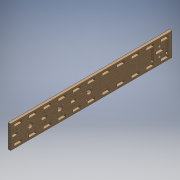
# Autodesk Inventor part: BearingMotorColumn
Saved by Autodesk Inventor 2016 (Build 200138000, 138)
## iProperties
Created: 2015-11-25
Part Number: BearingMotorColumn
Material: MDF Medium Density Fiberboard
Document SubType Name: Modeling
Designer: momem
Density: 0.8 g/cm^3
Appearance: Cardboard - Corrugated
MotorWidth: 37.000 mm
SupportClearance: 5.000 mm
MotorShaftWidth: 12.000 mm
CouplingWidth: 0.375 in
CouplingDiameter: 0.870 in
DiskGap: 75.835 mm
d28: 360.00 deg
ColumnWidth: 59.780 mm
WoodThickness: 6.390 mm
ColumnHeight: 417.094 mm
BearingDiameter: 24.000 mm
BearingWidth: 7.000 mm
BearingShaftDiameter: 8.000 mm
ZipTieWidth: 2.500 mm
ZipTieThickness: 1.100 mm
ZipTieClearance: 1.000 mm
ZipTieDistance: 10.000 mm
BearingHolderHeight: 13.100 mm
ZipTieHorDistance: 21.100 mm
ZipTieVerDistance: 9.500 mm
d97: 63.266 mm
d98: 227.506 mm
MotorWheel: 45.445 mm
BearingShaftOffset: 1.574 mm
BearingHolderHeight_1: 23.674 mm
LatchHeight: 13.147 mm
d176: 34.539 mm
Author: momem
Autodesk Inventor part; units mm, degrees
ref_plane "YZ Plane" through (0, 0, 0) normal (1, 0, 0) x (0, 1, 0)
ref_plane "XZ Plane" through (0, 0, 0) normal (0, 1, 0) x (-1, 0, 0)
ref_plane "XY Plane" through (0, 0, 0) normal (0, 0, 1) x (1, 0, 0)
sketch "Sketch1" plane through (0, 0, 0) normal (1, 0, 0) x (0, 1, 0)
  line L0 (37.9177, 29.89) -> (-37.9177, 29.89)
  line L1 (-37.9177, 29.89) -> (-37.9177, -29.89)
  line L2 (-37.9177, -29.89) -> (37.9177, -29.89)
  line L3 (37.9177, -29.89) -> (37.9177, 29.89) construction
  circle A0 centre (13.7687, 0) radius 6
  line L4 (-20.7703, 3.163) -> (-33.9177, 3.163)
  line L5 (-33.9177, 3.163) -> (-33.9177, -3.163)
  line L6 (-33.9177, -3.163) -> (-20.7703, -3.163)
  line L7 (-20.7703, -3.163) -> (-20.7703, 3.163)
  circle A1 centre (13.7687, 0) radius 11.049 construction
  circle A2 centre (6.7687, 0) radius 18.5 construction
  line L8 (28.4382, 24.8261) -> (9.4794, 24.8261)
  line L9 (9.4794, 24.8261) -> (9.4794, 18.5)
  line L10 (9.4794, 18.5) -> (28.4382, 18.5)
  line L11 (28.4382, 18.5) -> (28.4382, 24.8261)
  line L12 (-9.4794, 18.5) -> (-9.4794, 24.8261)
  line L13 (-9.4794, 24.8261) -> (-28.4382, 24.8261)
  line L14 (-28.4382, 18.5) -> (-9.4794, 18.5)
  line L15 (-28.4382, 24.8261) -> (-28.4382, 18.5)
  line L16 (28.4382, -24.89) -> (28.4382, -18.5639)
  line L17 (28.4382, -18.5639) -> (9.4794, -18.5639)
  line L18 (9.4794, -24.89) -> (28.4382, -24.89)
  line L19 (9.4794, -18.5639) -> (9.4794, -24.89)
  line L20 (-9.4794, -24.89) -> (-9.4794, -18.5639)
  line L21 (-9.4794, -18.5639) -> (-28.4382, -18.5639)
  line L22 (-28.4382, -24.89) -> (-9.4794, -24.89)
  line L23 (-28.4382, -18.5639) -> (-28.4382, -24.89)
  circle A3 centre (6.7687, -15.5) radius 1.5
  circle A4 centre (20.1921, -7.75) radius 1.5
  circle A5 centre (20.1921, 7.75) radius 1.5
  circle A6 centre (6.7687, 15.5) radius 1.5
  circle A7 centre (-6.6547, 7.75) radius 1.5
  circle A8 centre (-6.6547, -7.75) radius 1.5
  line L24 (-22.7703, 11.1) -> (-25.2703, 11.1)
  line L25 (-25.2703, 11.1) -> (-25.2703, 10)
  line L26 (-25.2703, 10) -> (-22.7703, 10)
  line L27 (-22.7703, 10) -> (-22.7703, 11.1)
  line L28 (-27.344, 3.1631) -> (-27.344, -3.1631) construction
  line L29 (-20.7703, 0) -> (-33.9177, 0) construction
  line L30 (-31.9177, 11.1) -> (-29.4177, 11.1)
  line L31 (-29.4177, 11.1) -> (-29.4177, 10)
  line L32 (-29.4177, 10) -> (-31.9177, 10)
  line L33 (-31.9177, 10) -> (-31.9177, 11.1)
  line L34 (-22.7703, -11.1) -> (-25.2703, -11.1)
  line L35 (-25.2703, -11.1) -> (-25.2703, -10)
  line L36 (-25.2703, -10) -> (-22.7703, -10)
  line L37 (-22.7703, -10) -> (-22.7703, -11.1)
  line L38 (-29.4177, -10) -> (-31.9177, -10)
  line L39 (-31.9177, -10) -> (-31.9177, -11.1)
  line L40 (-31.9177, -11.1) -> (-29.4177, -11.1)
  line L41 (-29.4177, -11.1) -> (-29.4177, -10)
  line L42 (315.9101, 29.89) -> (315.9101, -29.89) construction
  line L43 (331.7795, 14.945) -> (325.3895, 14.945)
  line L44 (325.3895, 14.945) -> (325.3895, -14.945)
  line L45 (325.3895, -14.945) -> (331.7795, -14.945)
  line L46 (331.7795, -14.945) -> (331.7795, 14.945)
  line L47 (315.9101, 29.89) -> (379.1766, 29.89)
  line L48 (379.1766, 29.89) -> (379.1766, -29.89)
  line L49 (379.1766, -29.89) -> (315.9101, -29.89)
  line L50 (357.0228, 3.195) -> (338.0639, 3.195)
  line L51 (338.0639, 3.195) -> (338.0639, -3.195)
  line L52 (338.0639, -3.195) -> (357.0228, -3.195)
  line L53 (357.0228, -3.195) -> (357.0228, 3.195)
  line L54 (347.5433, 29.89) -> (347.5433, -29.89) construction
  circle A9 centre (82.604, -15.5) radius 1.5
  line L55 (85.3147, -18.5639) -> (85.3147, -24.89)
  circle A10 centre (89.604, 0) radius 6
  line L56 (104.2736, -18.5639) -> (85.3147, -18.5639)
  line L57 (104.2736, -24.89) -> (104.2736, -18.5639)
  line L58 (85.3147, -24.89) -> (104.2736, -24.89)
  circle A11 centre (89.604, 0) radius 11.049 construction
  line L59 (85.3147, 18.5) -> (104.2736, 18.5)
  line L60 (104.2736, 24.8261) -> (85.3147, 24.8261)
  circle A12 centre (82.604, 0) radius 18.5 construction
  line L61 (55.065, -3.163) -> (55.065, 3.163)
  line L62 (50.565, -11.1) -> (50.565, -10)
  line L63 (50.565, -10) -> (53.065, -10)
  line L64 (53.065, -11.1) -> (50.565, -11.1)
  line L65 (53.065, -10) -> (53.065, -11.1)
  circle A13 centre (96.0274, -7.75) radius 1.5
  line L66 (66.3559, -24.89) -> (66.3559, -18.5639)
  line L67 (66.3559, -18.5639) -> (47.3971, -18.5639)
  line L68 (47.3971, -24.89) -> (66.3559, -24.89)
  line L69 (47.3971, -18.5639) -> (47.3971, -24.89)
  circle A14 centre (69.1806, -7.75) radius 1.5
  line L70 (85.3147, 24.8261) -> (85.3147, 18.5)
  line L71 (66.3559, 18.5) -> (66.3559, 24.8261)
  line L72 (66.3559, 24.8261) -> (47.3971, 24.8261)
  line L73 (47.3971, 18.5) -> (66.3559, 18.5)
  line L74 (47.3971, 24.8261) -> (47.3971, 18.5)
  circle A15 centre (82.604, 15.5) radius 1.5
  circle A16 centre (69.1806, 7.75) radius 1.5
  line L75 (50.565, 11.1) -> (50.565, 10)
  line L76 (53.065, 11.1) -> (50.565, 11.1)
  line L77 (53.065, 10) -> (53.065, 11.1)
  line L78 (50.565, 10) -> (53.065, 10)
  line L79 (48.4913, 3.163) -> (48.4913, -3.163) construction
  line L80 (55.065, 3.163) -> (41.9177, 3.163)
  line L81 (41.9177, -3.163) -> (55.065, -3.163)
  line L82 (55.065, 0) -> (41.9177, 0) construction
  line L83 (46.4177, -11.1) -> (46.4177, -10)
  line L84 (43.9177, -11.1) -> (46.4177, -11.1)
  line L85 (43.9177, -10) -> (43.9177, -11.1)
  line L86 (46.4177, -10) -> (43.9177, -10)
  line L87 (41.9177, 3.163) -> (41.9177, -3.163)
  line L88 (46.4177, 11.1) -> (46.4177, 10)
  line L89 (46.4177, 10) -> (43.9177, 10)
  line L90 (43.9177, 10) -> (43.9177, 11.1)
  line L91 (43.9177, 11.1) -> (46.4177, 11.1)
  line L92 (104.2736, 18.5) -> (104.2736, 24.8261)
  circle A17 centre (96.0274, 7.75) radius 1.5
  circle A18 centre (158.4393, -15.5) radius 1.5
  line L93 (161.15, -18.5639) -> (161.15, -24.89)
  circle A19 centre (165.4393, 0) radius 6
  line L94 (180.1089, -18.5639) -> (161.15, -18.5639)
  line L95 (180.1089, -24.89) -> (180.1089, -18.5639)
  line L96 (161.15, -24.89) -> (180.1089, -24.89)
  circle A20 centre (165.4393, 0) radius 11.049 construction
  line L97 (161.15, 18.5) -> (180.1089, 18.5)
  line L98 (180.1089, 24.8261) -> (161.15, 24.8261)
  circle A21 centre (158.4393, 0) radius 18.5 construction
  line L99 (130.9003, -3.163) -> (130.9003, 3.163)
  line L100 (126.4003, -11.1) -> (126.4003, -10)
  line L101 (126.4003, -10) -> (128.9003, -10)
  line L102 (128.9003, -11.1) -> (126.4003, -11.1)
  line L103 (128.9003, -10) -> (128.9003, -11.1)
  circle A22 centre (171.8627, -7.75) radius 1.5
  line L104 (142.1912, -24.89) -> (142.1912, -18.5639)
  line L105 (142.1912, -18.5639) -> (123.2324, -18.5639)
  line L106 (123.2324, -24.89) -> (142.1912, -24.89)
  line L107 (123.2324, -18.5639) -> (123.2324, -24.89)
  circle A23 centre (145.0159, -7.75) radius 1.5
  line L108 (161.15, 24.8261) -> (161.15, 18.5)
  line L109 (142.1912, 18.5) -> (142.1912, 24.8261)
  line L110 (142.1912, 24.8261) -> (123.2324, 24.8261)
  line L111 (123.2324, 18.5) -> (142.1912, 18.5)
  line L112 (123.2324, 24.8261) -> (123.2324, 18.5)
  circle A24 centre (158.4393, 15.5) radius 1.5
  circle A25 centre (145.0159, 7.75) radius 1.5
  line L113 (126.4003, 11.1) -> (126.4003, 10)
  line L114 (128.9003, 11.1) -> (126.4003, 11.1)
  line L115 (128.9003, 10) -> (128.9003, 11.1)
  line L116 (126.4003, 10) -> (128.9003, 10)
  line L117 (124.3266, 3.163) -> (124.3266, -3.163) construction
  line L118 (130.9003, 3.163) -> (117.753, 3.163)
  line L119 (117.753, -3.163) -> (130.9003, -3.163)
  line L120 (130.9003, 0) -> (117.753, 0) construction
  line L121 (122.253, -11.1) -> (122.253, -10)
  line L122 (119.753, -11.1) -> (122.253, -11.1)
  line L123 (119.753, -10) -> (119.753, -11.1)
  line L124 (122.253, -10) -> (119.753, -10)
  line L125 (117.753, 3.163) -> (117.753, -3.163)
  line L126 (122.253, 11.1) -> (122.253, 10)
  line L127 (122.253, 10) -> (119.753, 10)
  line L128 (119.753, 10) -> (119.753, 11.1)
  line L129 (119.753, 11.1) -> (122.253, 11.1)
  line L130 (180.1089, 18.5) -> (180.1089, 24.8261)
  circle A26 centre (171.8627, 7.75) radius 1.5
  line L131 (37.9177, 29.89) -> (189.5883, 29.89)
  line L132 (37.9177, -29.89) -> (189.5883, -29.89)
  line L133 (189.5883, 29.89) -> (315.9101, 29.89)
  line L134 (189.5883, -29.89) -> (315.9101, -29.89)
  line L135 (189.5883, 29.89) -> (189.5883, -29.89) construction
  line L136 (199.0677, -24.89) -> (218.0265, -24.89)
  line L137 (218.0265, -24.89) -> (218.0265, -18.5639)
  line L138 (218.0265, -18.5639) -> (199.0677, -18.5639)
  line L139 (199.0677, -18.5639) -> (199.0677, -24.89)
  line L140 (199.0677, 18.5) -> (218.0265, 18.5)
  line L141 (218.0265, 18.5) -> (218.0265, 24.8261)
  line L142 (218.0265, 24.8261) -> (199.0677, 24.8261)
  line L143 (199.0677, 24.8261) -> (199.0677, 18.5)
  line L144 (236.9854, -24.89) -> (255.9442, -24.89)
  line L145 (255.9442, -24.89) -> (255.9442, -18.5639)
  line L146 (255.9442, -18.5639) -> (236.9854, -18.5639)
  line L147 (236.9854, -18.5639) -> (236.9854, -24.89)
  line L148 (236.9854, 18.5) -> (255.9442, 18.5)
  line L149 (255.9442, 18.5) -> (255.9442, 24.8261)
  line L150 (255.9442, 24.8261) -> (236.9854, 24.8261)
  line L151 (236.9854, 24.8261) -> (236.9854, 18.5)
  line L152 (274.903, -24.89) -> (293.8619, -24.89)
  line L153 (293.8619, -24.89) -> (293.8619, -18.5639)
  line L154 (293.8619, -18.5639) -> (274.903, -18.5639)
  line L155 (274.903, -18.5639) -> (274.903, -24.89)
  line L156 (274.903, 18.5) -> (293.8619, 18.5)
  line L157 (293.8619, 18.5) -> (293.8619, 24.8261)
  line L158 (293.8619, 24.8261) -> (274.903, 24.8261)
  line L159 (274.903, 24.8261) -> (274.903, 18.5)
  line L160 (312.8207, -24.89) -> (331.7795, -24.89)
  line L161 (331.7795, -24.89) -> (331.7795, -18.5639)
  line L162 (331.7795, -18.5639) -> (312.8207, -18.5639)
  line L163 (312.8207, -18.5639) -> (312.8207, -24.89)
  line L164 (312.8207, 18.5) -> (331.7795, 18.5)
  line L165 (331.7795, 18.5) -> (331.7795, 24.8261)
  line L166 (331.7795, 24.8261) -> (312.8207, 24.8261)
  line L167 (312.8207, 24.8261) -> (312.8207, 18.5)
  line L168 (350.7383, -24.89) -> (369.6972, -24.89)
  line L169 (369.6972, -24.89) -> (369.6972, -18.5639)
  line L170 (369.6972, -18.5639) -> (350.7383, -18.5639)
  line L171 (350.7383, -18.5639) -> (350.7383, -24.89)
  line L172 (350.7383, 18.5) -> (369.6972, 18.5)
  line L173 (369.6972, 18.5) -> (369.6972, 24.8261)
  line L174 (369.6972, 24.8261) -> (350.7383, 24.8261)
  line L175 (350.7383, 24.8261) -> (350.7383, 18.5)
  line L176 (363.3072, 14.945) -> (369.6972, 14.945)
  line L177 (369.6972, 14.945) -> (369.6972, -14.945)
  line L178 (369.6972, -14.945) -> (363.3072, -14.945)
  line L179 (363.3072, -14.945) -> (363.3072, 14.945)
  circle A27 centre (-27.344, 0) radius 12 construction
  line L180 (-8.954, 29.89) -> (-8.954, -29.89) construction
  circle A28 centre (13.7687, 0) radius 22.7227 construction
  line L181 (-9.4794, 21.663) -> (-28.4382, 21.663) construction
  line L182 (-18.9588, 24.8261) -> (-18.9588, 18.5) construction
  line L183 (366.5022, 14.945) -> (366.5022, -14.945) construction
  circle A29 centre (347.5433, 11.6113) radius 3.3337
  circle A30 centre (347.5433, -11.6113) radius 3.3337
  point P0 (0, 0)
  point P1 (37.9177, 0)
  point P2 (0, -29.89)
  point P3 (357.0228, 0)
  point P4 (379.1766, 0)
  point P5 (347.5433, -3.195)
  point P6 (325.3895, 0)
  point P7 (315.9101, 0)
  point P8 (-27.344, 0)
  point P9 (360.2178, 24.8261)
  dimension "ColumnWidth" = 59.78
  dimension "d1" = 12
  dimension "d2" = 13.1473
  dimension "d3" = 6.3261
  dimension "d4" = 4
  dimension "d5" = 22.098
  dimension "d6" = 34.539
  dimension "d8" = 37
  dimension "d9" = 7
  dimension "DiskGap" = 75.8353
  dimension "d12" = 18.9588
  dimension "d13" = 6.3261
  dimension "d14" = 9.4794
  dimension "d17" = 37.9177
  dimension "d20" = 43.39
  dimension "d23" = 3
  dimension "d24" = 15.5
  dimension "d28" = 360
  dimension "d32" = 2.5
  dimension "d33" = 1.1
  dimension "d34" = 2
  dimension "d35" = 10
  dimension "d77" = 24.149
  dimension "d78" = 29.89
  dimension "d80" = 6.39
  dimension "d81" = 9.4794
  dimension "d83" = 18.9588
  dimension "d84" = 6.39
  dimension "ColumnHeight" = 417.0942
  dimension "d89" = 75.8353
  dimension "d94" = 151.6706
  dimension "d97" = 63.2665
  dimension "d98" = 227.506
  dimension "d103" = 37.9177
  dimension "d112" = 24
  dimension "d113" = 0
  dimension "d116" = 18.39
  dimension "MotorWheel" = 45.4453
  dimension "d170" = 6.6675
  dimension "d176" = 34.539
  constraints: 368 end point, 31 centre point, 21 midpoint, 17 symmetric about line, 13 horizontal, 13 parallel, 9 perpendicular, 6 horizontal alignment, 5 coincident, 5 collinear, 4 vertical alignment, 3 point on line, 3 tangent, 3 vertical, 307 other
  measures "ColumnWidth" distance of L2.end L0.start
  measures "d1" diameter of A0
  measures "d2" distance of L6.end L5.end
  measures "d3" distance of L6.end L4.start
  measures "d4" distance between parallel lines of L1 L5
  measures "d5" diameter of A1
  measures "d6" distance from line of L7 A1.centre
  measures "d8" diameter of A2
  measures "d9" distance of A2.centre A1.centre
  measures "DiskGap" distance between parallel lines of L1 L3
  measures "d12" distance of L8.start L8.end
  measures "d13" distance of L10.end L8.start
  measures "d14" distance between parallel lines of L3 L11
  measures "d17" distance of L10.end L12.start
  measures "d20" distance of L10.end L16.start
  measures "d23" diameter of A3
  measures "d24" distance of A2.centre A3.centre
  measures "d32" distance of L24.start L24.end
  measures "d33" distance of L24.end L25.end
  measures "d34" distance between parallel lines of L7 L27
  measures "d35" distance from line of L29.start L26
  measures "d77" distance from line of L3 A0.centre
  measures "d78" distance of L45.end L43.start
  measures "d80" distance of L43.start L43.end
  measures "d81" distance between parallel lines of L42 L44
  measures "d83" distance between parallel lines of L51 L53
  measures "d84" distance of L52.end L50.start
  measures "ColumnHeight" distance between parallel lines of L1 L48
  measures "d89" distance of A3.centre A9.centre
  measures "d94" distance of L0.start L131.end
  measures "d97" distance of L48.end L42.end
  measures "d98" distance between parallel lines of L1 L135
  measures "d103" distance of L93.end L136.start
  measures "d112" diameter of A27
  measures "d113" distance from line of L28 A27.centre
  measures "d116" distance from line of A27.centre L180
  measures "MotorWheel" diameter of A28
  measures "d170" diameter of A29
  measures "d176" distance from line of A0.centre L7
extrude "Extrusion8" add sketch "Sketch1" along normal blind 6.39
equation "\"ColumnWidth\" = 2 * WoodThickness + MotorWidth + 2 * SupportClearance"
equation "\"d1\" = MotorShaftWidth"
equation "\"d4\" = 0.166667 * BearingDiameter"
equation "\"d5\" = CouplingDiameter"
equation "\"d6\" = BearingHolderHeight + 0.166667 * BearingDiameter + 0.5 * CouplingDiameter + WoodThickness"
equation "\"d8\" = MotorWidth"
equation "\"d12\" = 0.25 * DiskGap"
equation "\"d14\" = 0.125 * DiskGap"
equation "\"d17\" = 0.5 * DiskGap"
equation "\"d20\" = MotorWidth + WoodThickness"
equation "\"d32\" = ZipTieWidth"
equation "\"d33\" = ZipTieThickness"
equation "\"d34\" = 2 * ZipTieClearance"
equation "\"d77\" = 0.5 * CouplingDiameter + BearingHolderHeight"
equation "\"MotorWidth\" = 37"
equation "\"SupportClearance\" = 5"
equation "\"MotorShaftWidth\" = 12"
equation "\"CouplingWidth\" = 9.525"
equation "\"CouplingDiameter\" = 22.098"
equation "\"BearingHolderHeight\" = 13.1"
equation "\"ZipTieHorDistance\" = 21.1"
equation "\"ZipTieVerDistance\" = 9.5"
equation "\"WoodThickness\" = 6.39"
equation "\"BearingDiameter\" = 24"
equation "\"ZipTieWidth\" = 2.5"
equation "\"ZipTieThickness\" = 1.1"
equation "\"ZipTieClearance\" = 1"
body "Solid7"
